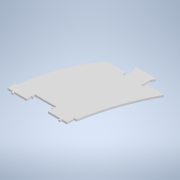
# Autodesk Inventor part: Support C
Saved by Autodesk Inventor 2020 (Build 240168000, 168)
## iProperties
Created: 2020-03-07
Part Number: Support C
Material: Generic
Document SubType Name: Modeling
Designer: Daniel Wikman
Density: 1 g/cm^3
Appearance: Default
Author: Daniel Wikman
Autodesk Inventor part; units mm, degrees
ref_plane "YZ Plane" through (0, 0, 0) normal (1, 0, 0) x (0, 1, 0)
ref_plane "XZ Plane" through (0, 0, 0) normal (0, 1, 0) x (-1, 0, 0)
ref_plane "XY Plane" through (0, 0, 0) normal (0, 0, 1) x (1, 0, 0)
sketch "Sketch1" plane through (0, 0, 0) normal (0, 1, 0) x (-1, 0, 0)
  line L0 (113.8016, -163.8079) -> (118.6285, -172.1682)
  line L1 (113.8016, -163.8079) -> (118.4883, -163.8079)
  arc A0 (32.1771, -413.0024) -> (33.3318, -411.0024) centre (32.1771, -411.669) ccw
  line L2 (26.4886, -397.8099) -> (26.4886, -373.629)
  arc A1 (26.4886, -370.9624) -> (26.4886, -373.629) centre (26.4886, -372.2957) ccw
  line L3 (26.4886, -370.9624) -> (32.9886, -370.9624)
  arc A2 (32.9886, -373.629) -> (32.9886, -370.9624) centre (32.9886, -372.2957) ccw
  line L4 (32.9886, -373.629) -> (32.9886, -380.9624)
  line L5 (-88.7072, -380.9624) -> (-33.5061, -380.9624)
  line L6 (32.9886, -380.9624) -> (90.3221, -380.9624)
  arc A3 (-33.9776, -411.0024) -> (-32.8229, -413.0024) centre (-32.8229, -411.669) ccw
  arc A4 (-27.1344, -373.6228) -> (-27.0061, -370.9624) centre (-27.0061, -372.2957) ccw
  line L7 (-27.0061, -370.9624) -> (-33.5061, -370.9624)
  arc A5 (-33.5061, -370.9624) -> (-33.5061, -373.629) centre (-33.5061, -372.2957) ccw
  line L8 (-33.5061, -373.629) -> (-33.5061, -380.9624)
  line L9 (118.4883, -148.1364) -> (118.4883, -161.1412)
  line L10 (33.3318, -411.0024) -> (27.1585, -400.3099)
  arc A6 (26.4886, -397.8099) -> (27.1585, -400.3099) centre (31.4886, -397.8099) ccw
  line L11 (-27.1344, -397.8099) -> (-27.1344, -373.6228)
  line L12 (-33.9776, -411.0024) -> (-27.8043, -400.3099)
  arc A7 (-27.8043, -400.3099) -> (-27.1344, -397.8099) centre (-32.1344, -397.8099) ccw
  line L13 (-32.8229, -413.0024) -> (32.1771, -413.0024)
  line L14 (-11.4601, -148.0629) -> (-11.4601, -168.7264)
  line L15 (156.6836, -142.6364) -> (162.6836, -142.6364)
  line L16 (162.6836, -142.6364) -> (162.6836, -148.1364)
  line L17 (156.6866, -148.1364) -> (118.4883, -148.1364)
  line L18 (11.6836, -145.4697) -> (11.6846, -142.6364)
  line L19 (11.6846, -142.6364) -> (5.6846, -142.6364)
  line L20 (5.6846, -142.6364) -> (5.6845, -148.1281)
  line L21 (11.6831, -148.1364) -> (49.8814, -148.1364)
  arc A8 (11.6836, -145.4697) -> (11.6831, -148.1364) centre (11.6831, -146.803) ccw
  arc A9 (3.0194, -148.0629) -> (5.6845, -148.1281) centre (4.3512, -148.1281) ccw
  line L22 (-11.4601, -148.0629) -> (3.0194, -148.0629)
  line L23 (-11.4601, -171.393) -> (-18.9601, -171.393)
  arc A10 (-11.4601, -171.393) -> (-11.4601, -168.7264) centre (-11.4601, -170.0597) ccw
  line L24 (162.6836, -145.3864) -> (185.043, -145.3864) construction
  line L25 (21.6753, -413.0028) -> (-28.7481, -413.0028) construction
  line L26 (-0.3229, -413.0028) -> (-0.3229, -413.0028)
  arc A11 (-89.9069, -379.0472) -> (-88.7072, -380.9624) centre (-88.7072, -379.629) ccw
  line L27 (156.6836, -142.6364) -> (156.6836, -145.4697)
  line L28 (165.3503, -148.1364) -> (179.8299, -148.1364)
  arc A12 (156.6866, -148.1364) -> (156.6836, -145.4697) centre (156.6836, -146.803) ccw
  arc A13 (162.6836, -148.1364) -> (165.3503, -148.1364) centre (164.017, -148.1364) ccw
  line L29 (179.8299, -148.1364) -> (179.8299, -171.4697)
  line L30 (179.8299, -171.4697) -> (172.3299, -171.4697)
  line L31 (90.3221, -380.9624) -> (90.3221, -378.9624)
  line L32 (90.3221, -376.2957) -> (97.8221, -376.2957)
  arc A14 (90.3221, -376.2957) -> (90.3221, -378.9624) centre (90.3221, -377.629) ccw
  line L33 (118.4883, -161.1412) -> (118.4883, -164.2811)
  arc A15 (118.4883, -163.8079) -> (118.4883, -161.1412) centre (118.4883, -162.4745) ccw
  line L34 (84.1849, -148.1364) -> (84.1849, -155.2534)
  arc A16 (117.4738, -174.1682) -> (118.6285, -172.1682) centre (117.4738, -172.8349) ccw
  line L35 (84.1849, -174.1682) -> (117.4738, -174.1682)
  line L36 (54.5681, -163.8079) -> (49.7413, -172.1682)
  line L37 (54.5681, -163.8079) -> (49.8814, -163.8079)
  line L38 (49.8814, -148.1364) -> (49.8814, -161.1412)
  line L39 (49.8814, -161.1412) -> (49.8814, -164.2811)
  arc A17 (49.8814, -161.1412) -> (49.8814, -163.8079) centre (49.8814, -162.4745) ccw
  arc A18 (49.7413, -172.1682) -> (50.896, -174.1682) centre (50.896, -172.8349) ccw
  line L40 (84.1849, -174.1682) -> (50.896, -174.1682)
  arc A19 (97.8221, -376.2957) -> (172.3299, -171.4697) centre (-250.9666, -133.4553) ccw
  arc A20 (-89.9069, -379.0472) -> (-18.9601, -171.393) centre (-669.0585, -65.2283) ccw
  point P0 (-90.8396, -380.9624)
  point P1 (-27.3048, -399.1039)
  dimension "d102" = 2.6667
  dimension "d107" = 2.6667
  dimension "d108" = 6.5
  dimension "d109" = 2.6667
  dimension "d141" = 7.3333
  dimension "d142" = 5
  dimension "d170" = 13.0048
  dimension "d173" = 6
  dimension "d174" = 5.5
  dimension "d177" = 7.5
  dimension "d179" = 2.6667
  dimension "d181" = 232.826
  dimension "d183" = 264.8664
  dimension "d184" = 23.3301
  dimension "d186" = 57.3335
  dimension "d187" = 57.3335
  dimension "d189" = 6.5
  dimension "d190" = 7.3333
  dimension "d191" = 24.187
  dimension "d192" = 1.3333
  dimension "d202" = 6
  dimension "d203" = 1.3333
  dimension "d204" = 1.3333
  dimension "d208" = 191.29
  dimension "d209" = 2.6667
  dimension "d210" = 2.6667
  dimension "d211" = 14.4796
  dimension "d212" = 14.4796
  dimension "d213" = 61.3416
  dimension "d214" = 145
  dimension "d216" = 23.3333
  dimension "d217" = 7.5
  dimension "d220" = 7.5
  dimension "d221" = 2.6667
  dimension "d223" = 38.1984
  dimension "d226" = 61.3416
  dimension "d232" = 2.6667
  dimension "d233" = 2.6667
  dimension "d234" = 61.3416
  dimension "d235" = 60
  dimension "d236" = 33.2889
  dimension "d237" = 2
  dimension "d238" = 425
  dimension "d239" = 658.71
  constraints: 83 end point, 44 point on circle, 21 centre point, 13 point on line, 12 horizontal, 9 vertical, 8 symmetric about line, 8 tangent, 2 collinear, 2 equal length, 1 midpoint, 1 perpendicular, 11 other
  measures "d102" diameter of A0
  measures "d107" diameter of A1
  measures "d108" distance of L3.start L3.end
  measures "d109" diameter of A2
  measures "d141" distance of L4.start L4.end
  measures "d142" radius of A6
  measures "d170" distance of L9.start L9.end
  measures "d173" distance of L15.start L15.end
  measures "d174" distance of L16.end L15.end
  measures "d177" distance of L23.start L23.end
  measures "d179" diameter of A10
  measures "d181" vertical distance of L5.end L21.end
  measures "d183" distance between parallel lines of L21 L25
  measures "d184" distance between parallel lines of L23 L22
  measures "d186" distance of point (-90.84, -380.962) L5.end
  measures "d187" distance of L4.end L6.end
  measures "d189" distance of L7.start L7.end
  measures "d190" distance of L8.start L5.end
  measures "d191" distance of L11.start L11.end
  measures "d192" radius of A11
  measures "d202" distance of L18.end L19.end
  measures "d203" radius of A8
  measures "d204" radius of A9
  measures "d208" distance of L14.start L28.end
  measures "d209" diameter of A12
  measures "d210" diameter of A13
  measures "d211" distance of L28.start L28.end
  measures "d212" distance of L14.start L22.end
  measures "d213" distance from line of L28.end L9
  measures "d214" distance from line of L18.start L27
  measures "d216" distance of L28.end L29.end
  measures "d217" distance of L29.end L30.end
  measures "d220" distance of L32.start L32.end
  measures "d221" diameter of A14
  measures "d223" distance of L21.start L21.end
  measures "d226" distance of L21.end L14.start
  measures "d232" diameter of A15
  measures "d233" diameter of A16
  measures "d234" distance from line of L14 L21.end
  measures "d235" angle of L35 L0
  measures "d236" distance of L35.start L35.end
  measures "d237" distance of L6.end L31.end
  measures "d238" radius of A19
  measures "d239" radius of A20
extrude "Extrusion4" add sketch "Sketch1" along normal blind 6 contours L1 A15 L9 L17 A12 L27 L15 L16 A13 L28 L29 L30 A19 L32 A14 L31 L6 L4 A2 L3 A1 L2 A6 L10 A0 L13 A3 L12 A7 L11 A4 L7 A5 L8 L5 A11 A20 L23 A10 L14 L22 A9 L20 L19 L18 A8 L21 L38 A17 L37 L36 A18 L40 L35 A16 L0
body "Solid4"
